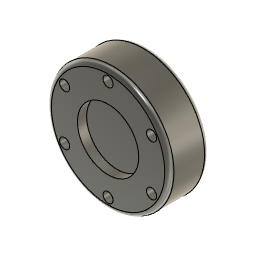
7-rolima (Autodesk Fusion 360 design; units mm, degrees)
Autodesk Fusion 360 part; units mm, degrees
sketch "Sketch1" plane through (0, 0, 0) normal (0, 1, 0) x (1, 0, 0)
  circle A0 centre (0, 0) radius 10
  circle A1 centre (0, 0) radius 20
  circle A2 centre (0, 0) radius 18.0278 construction
  circle A3 centre (-0.0049, -16.3778) radius 1.65
  line L0 (0, -22) -> (0, 22) construction
  line L1 (-25, 0) -> (28, 0) construction
  circle A4 centre (0, 0) radius 10
  circle A5 centre (0, 0) radius 10
  circle A6 centre (14.1811, -8.1931) radius 1.65
  circle A7 centre (14.186, 8.1846) radius 1.65
  circle A8 centre (0.0049, 16.3778) radius 1.65
  circle A9 centre (-14.1811, 8.1931) radius 1.65
  circle A10 centre (-14.186, -8.1846) radius 1.65
  point P0 (-0.0049, -16.3778)
  point P1 (-0.0049, 16.3778)
  dimension "d1" = 20
  dimension "d2" = 40
  dimension "d3" = 3.3
  dimension "d16" = 360
  constraint coincident A0.centre A1.centre
  constraint concentric A1 A2
  constraint tangent A2 A3
  constraint vertical L0
  constraint horizontal L1
  constraint symmetric A0 L1 A4
  constraint symmetric L1 A4 A5
  constraint coincident P0 A3.centre
  measures "d1" diameter of A0
  measures "d2" diameter of A1
  measures "d3" diameter of A3
extrude "Extrude1" add sketch "Sketch1" along normal blind 13 contours A0 A4 A5 | A1 | A3 | A6 | A7 | A8 | A9 | A10
extrude "Extrude3" cut sketch "Sketch1" along normal blind 3 contours A0 A4 A5
fillet "Fillet1" radius 1.5 2 edges at (-18.6465, 0, 7.2323) (-18.6465, 13, 7.2323)
extrude "Extrude4" cut sketch "Sketch1" along normal blind 8 contours A3 | A6 | A7 | A8 | A9 | A10
sketch "Sketch2" plane through (0, 13, 0) normal (0, 1, 0) x (-1, 0, 0)
  circle A0 centre (0, 0) radius 18.5
  circle A1 centre (0, 0) radius 18
  dimension "d17" = 36
  constraint concentric A0 A1
  measures "d17" diameter of A1
extrude "Extrude5" cut sketch "Sketch2" against normal blind 3 contours A1
